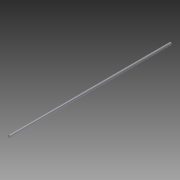
# Autodesk Inventor part: OCT_tubing_21G
Saved by Autodesk Inventor 2011 SP2 (Build 150309200, 309)
## iProperties
Created: 2012-04-17
Part Number: OCT_tubing_21G
Document SubType Name: Modeling
Designer: sungwook
Density: 1 g/cm^3
Author: sungwook
Autodesk Inventor part; units mm, degrees
ref_plane "YZ Plane" through (0, 0, 0) normal (1, 0, 0) x (0, 1, 0)
ref_plane "XZ Plane" through (0, 0, 0) normal (0, 1, 0) x (-1, 0, 0)
ref_plane "XY Plane" through (0, 0, 0) normal (0, 0, 1) x (1, 0, 0)
sketch "Sketch1" plane through (0, 0, 0) normal (0, 0, 1) x (1, 0, 0)
  circle A0 centre (0, 0) radius 0.254
  circle A1 centre (0, 0) radius 0.4064
  dimension "d0" = 0.508
  dimension "d1" = 0.8128
  constraints: 2 centre point, 2 coincident
  measures "d0" diameter of A0
  measures "d1" diameter of A1
extrude "Extrusion1" add sketch "Sketch1" along normal blind 53
equation "\"d2\" = OCTd0 - OCTd1"
equation "\"lOCT\" = 58"
equation "\"OCToffset\" = 14.38"
equation "\"lOCTprobeNom\" = 72.38"
equation "\"OCTd0\" = 73"
equation "\"OCTd1\" = 20"
body "Solid1"
